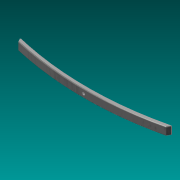
# Autodesk Inventor part: leaf 3
Saved by Autodesk Inventor 2014 SP2 (Build 180246200, 246)
## iProperties
Created: 2019-07-17
Part Number: leaf 3
Material: Steel, Carbon
Document SubType Name: Modeling
Designer: USER PC
Density: 7.87 g/cm^3
Appearance: Semi-Polished
Mass: 1961.93 g
Surface Area: 491.969 cm^2
Volume: 249.292 cm^3
Author: USER PC
Autodesk Inventor part; units mm, degrees
ref_plane "YZ Plane" through (0, 0, 0) normal (1, 0, 0) x (0, 1, 0)
ref_plane "XZ Plane" through (0, 0, 0) normal (0, 1, 0) x (-1, 0, 0)
ref_plane "XY Plane" through (0, 0, 0) normal (0, 0, 1) x (1, 0, 0)
sketch "Sketch1" plane through (0, 0, 0) normal (0, 0, 1) x (1, 0, 0)
  arc A0 (0.1634, -91.6592) -> (286.7211, -56.9812) centre (0.1634, 1109.6463) ccw
  arc A1 (0.1634, -106.6592) -> (276.3881, -74.8786) centre (0.1634, 1109.6463) ccw
  line L0 (286.7211, -56.9812) -> (276.3881, -74.8786)
  line L1 (286.7211, -56.9812) -> (307.3872, -56.9812) construction
  line L2 (0.1634, -106.6592) -> (0.1634, -82.9582)
  arc A2 (-286.3942, -56.9812) -> (0.1634, -91.6592) centre (0.1634, 1109.6463) ccw
  arc A3 (-276.0612, -74.8786) -> (0.1634, -106.6592) centre (0.1634, 1109.6463) ccw
  line L3 (-286.3942, -56.9812) -> (-276.0612, -74.8786)
  point P0 (0, 0)
  point P1 (254.828, -79.7002)
  dimension "d0" = 15
  dimension "d1" = 120
  constraints: 9 point on circle, 8 end point, 4 centre point, 2 symmetric about line, 1 equal length, 1 horizontal, 1 perpendicular, 2 other
  measures "d0" radial gap between concentric circles of A1 A0
  measures "d1" angle of L0 L1
extrude "Extrusion1" add sketch "Sketch1" along normal blind 30
fillet "Fillet1" radius 3 12 edges at (-144.1607, -82.9582, 30) (139.1869, -98.6879, 30) (144.4876, -82.9582, 0) (286.7211, -56.9812, 15) (281.5546, -65.9299, 0) (281.5546, -65.9299, 30) (276.3881, -74.8786, 15) (139.1869, -98.6879, 0) (-286.3942, -56.9812, 15) (-281.2277, -65.9299, 30) (-276.0612, -74.8786, 15) (-281.2277, -65.9299, 0)
sketch "Sketch2" plane through (0, 0, 0) normal (0, 1, 0) x (-1, 0, 0)
  line L0 (0, 0) -> (0, 15)
  circle A0 centre (0, 15) radius 5
  dimension "d5" = 15
  dimension "d6" = 10
  constraints: 2 end point, 1 centre point, 1 coincident, 1 vertical
  measures "d5" distance of L0.start L0.end
  measures "d6" diameter of A0
extrude "Extrusion2" cut sketch "Sketch2" against normal blind 300
body "Solid1"
